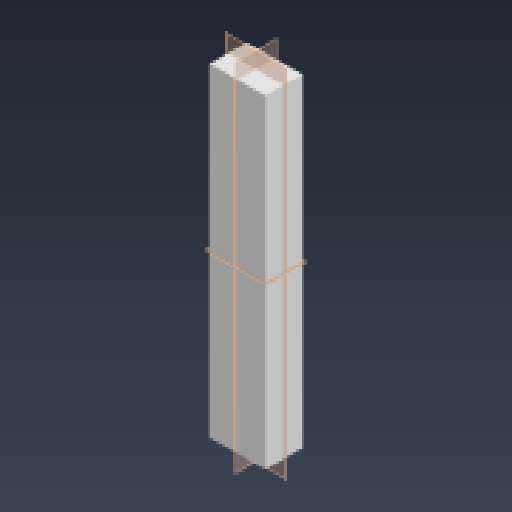
# Autodesk Inventor part: Направляющая
Saved by Autodesk Inventor 2023.2 (Build 272271030, 271C)
## iProperties
Created: 2026-01-04
Part Number: Направляющая
Material: Типовые
Document SubType Name: Modeling
Designer: Олег Коноваленко
Density: 1 g/cm^3
Appearance: По умолчанию
Author: Олег Коноваленко
Autodesk Inventor part; units mm, degrees
sketch "Эскиз1" plane through (0, 0, 0) normal (0, 1, 0) x (-1, 0, 0)
  line L0 (6, 4) -> (-6, 4)
  line L1 (-6, 4) -> (-6, -4)
  line L2 (-6, -4) -> (6, -4)
  line L3 (6, -4) -> (6, 4)
  line L4 (6, 4) -> (-6, -4) construction
  line L5 (-6, 4) -> (6, -4) construction
  point P0 (0, 0)
  dimension "d0" = 12
  dimension "d1" = 8
  constraints: 12 end point, 2 midpoint, 2 parallel, 1 horizontal, 1 perpendicular
  measures "d0" distance of L1.end L2.end
  measures "d1" distance of L0.end L1.end
extrude "Выдавливание1" add sketch "Эскиз1" along normal mid plane 50
